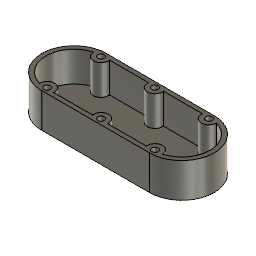
assembly_V.1 (Autodesk Fusion 360 archive; units mm, degrees)
design "robosoc_motor_case_without_motor_V.1"
part number: 2025-12-10-15-49-31-313
Autodesk Fusion 360 part; units mm, degrees
note: some values were not read from the file. Set by a fixed rule: the direction of a hole.
sketch "Sketch1" plane through (0, 0, 0) normal (0, 0, 1) x (1, 0, 0)
  line L0 (15, 0) -> (65, 0)
  line L1 (65, 30) -> (15, 30)
  arc A0 (15, 30) -> (0, 15) centre (15, 15) ccw
  arc A1 (0, 15) -> (15, 0) centre (15, 15) ccw
  arc A2 (80, 15) -> (65, 30) centre (65, 15) ccw
  arc A3 (65, 0) -> (80, 15) centre (65, 15) ccw
  line L2 (15, 15) -> (65, 15) construction
  line L3 (15, 15) -> (15, 27.5) construction
  line L4 (65, 15) -> (65, 27.5) construction
  line L5 (15, 27.5) -> (40, 27.5) construction
  circle A4 centre (15, 27.5) radius 1.5
  circle A5 centre (40, 27.5) radius 1.5
  circle A6 centre (65, 27.5) radius 1.5
  circle A7 centre (15, 2.5) radius 1.5
  circle A8 centre (40, 2.5) radius 1.5
  circle A9 centre (65, 2.5) radius 1.5
  circle A10 centre (65, 15) radius 2.5
  circle A11 centre (15, 15) radius 2.5
  point P0 (80, 0)
  point P1 (0, 30)
  dimension "d1" = 80
  dimension "d2" = 30
  dimension "d3" = 15
  dimension "d4" = 15
  dimension "d5" = 15
  dimension "d6" = 15
  dimension "d7" = 12.5
  dimension "d8" = 12.5
  dimension "d9" = 25
  dimension "d11" = 3
  dimension "d12" = 3
  dimension "d13" = 3
  dimension "d22" = 5
  dimension "d23" = 5
  constraint horizontal L0
  constraint horizontal L1
  constraint coincident P1 L1
  constraint tangent L1 A0
  constraint coincident origin L0
  constraint tangent L0 A1
  constraint coincident A0.end A1.start
  constraint tangent L1 A2
  constraint coincident P0 L0
  constraint tangent L0 A3
  constraint coincident A2.start A3.end
  constraint coincident A0.centre A1.centre
  constraint coincident A2.centre A3.centre
  constraint perpendicular L1 L3
  constraint perpendicular L2 L4
  constraint perpendicular L3 L5
  constraint coincident L3.end L5.start
  constraint coincident L5.end A5.centre
  constraint coincident L4.end A6.centre
  constraint symmetric L2 A4 A7
  constraint symmetric L2 A5 A8
  constraint symmetric L2 A6 A9
  constraint concentric A3 A10
  constraint concentric A1 A11
  measures "d1" distance of origin P0
  measures "d2" distance of origin P1
  measures "d3" radius of A0
  measures "d4" radius of A1
  measures "d5" radius of A2
  measures "d6" radius of A3
  measures "d7" distance of A0.centre L3.end
  measures "d8" distance of A2.centre L4.end
  measures "d9" distance of L3.end L5.end
  measures "d11" diameter of A4
  measures "d12" diameter of A5
  measures "d13" diameter of A6
  measures "d22" diameter of A10
  measures "d23" diameter of A11
extrude "Extrude1" add sketch "Sketch1" along normal blind 16 contours L0 L1 A0 A1 A2 A3 | A10 | A11
shell "Shell1" thickness 2 removed faces 1 at (23.6999, 18.8266, 16)
hole "Hole1" at (65, 27.5, 0) at (40, 27.5, 0) at (15, 27.5, 0) at (15, 2.5, 0) at (40, 2.5, 0) at (65, 2.5, 0) direction (0, 0, 1) diameter 4 depth 1 tip angle 180 countersink diameter 4.4 countersink angle 90
extrude "Extrude2" add sketch "Sketch1" against normal blind 4 draft -15 contours A10 | A11
equation "d23 = d22"

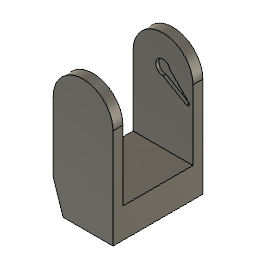
design "robosoc_leg_holder_V.1"
part number: 2025-12-04-10-49-25-755
Autodesk Fusion 360 part; units mm, degrees
sketch "Sketch1" plane through (0, 0, 0) normal (0, 1, 0) x (1, 0, 0)
  line L0 (5, 0) -> (30, 0)
  line L1 (30, 0) -> (30, -50)
  line L2 (0, -50) -> (0, -15)
  arc A0 (0, -50) -> (30, -50) centre (15, -50) ccw
  circle A1 centre (15, -50) radius 1.5
  line L3 (30, 0) -> (5, 0) construction
  line L4 (0, -15) -> (5, 0)
  line L5 (0, -15) -> (30, -15)
  dimension "d2" = 50
  dimension "d4" = 3
  dimension "d5" = 25
  dimension "d6" = 15
  dimension "d9" = 30
  constraint horizontal L0
  constraint vertical L1
  constraint vertical L2
  constraint concentric A0 A1
  constraint perpendicular L1 L3
  constraint perpendicular L1 L5
  measures "d2" distance of origin L2.start
  measures "d4" diameter of A1
  measures "d5" distance of L0.end L0.start
  measures "d6" distance of origin L2.end
  measures "d9" distance of L2.end L5.end
extrude "Extrude1" add sketch "Sketch1" along normal blind 5 contours L0 L1 L4 L5 | L1 L2 A0 L5 | A1
extrude "Extrude2" cut sketch "Sketch1" along normal blind 45 contours L0 L1 L4 L5
extrude "Extrude3" add sketch "Sketch1" along normal blind 22.5 contours L0 L1 L4 L5
mirror "Mirror1" about plane through (0, 22.5, 0) normal (0, 1, 0) of bodies 1 merged
hole "Hole2" at (15, 5, 50) direction (0, -1, 0) diameter 4.5 depth 4 tip angle 180
sketch "Sketch2" plane through (0, 40, 0) normal (0, -1, 0) x (1, 0, 0)
  line L0 (0, 15) -> (30, 15)
  line L1 (30, 15) -> (30, 50)
  arc A0 (30, 50) -> (0, 50) centre (15, 50) ccw
  line L2 (0, 50) -> (0, 15)
  line L3 (14.9863, 46.4) -> (18.4859, 50.8992) construction
  line L4 (15, 50) -> (28.0239, 39.8695) construction
  line L5 (18.4859, 50.8992) -> (27.951, 41.1812)
  line L6 (14.9863, 46.4) -> (26.7346, 39.6174)
  arc A1 (26.7346, 39.6174) -> (27.951, 41.1812) centre (27.2346, 40.4835) ccw
  arc A2 (18.4859, 50.8992) -> (14.9863, 46.4) centre (15, 50) ccw
  dimension "d24" = 7.2
  dimension "d25" = 2
  dimension "d26" = 5.7
  dimension "d28" = 16.5
  constraint concentric A0 A2
  constraint coincident A0.centre L4.start
  constraint coincident L4.end A1
  constraint tangent L5 A1
  constraint tangent L6 A1
  constraint perpendicular L3 L4
  constraint coincident A1.centre L4
  measures "d24" diameter of A2
  measures "d25" diameter of A1
  measures "d26" distance of L3.start L3.end
  measures "d28" distance of A0.centre L4.end
extrude "Extrude4" cut sketch "Sketch2" against normal blind 1.5 contours L5 L6 A1 A2
hole "Hole1" at (17.5, 22.5, 0) direction (0, 0, 1) diameter 19 depth 13 tip angle 180 countersink diameter 21 countersink angle 10

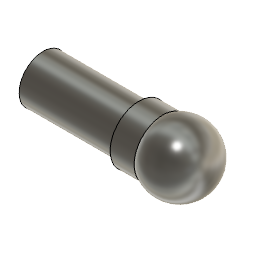
design "robosoc_leg_piece_V.1"
part number: 2025-12-04-11-27-23-377
Autodesk Fusion 360 part; units mm, degrees
sketch "Sketch1" plane through (0, 0, 0) normal (0, 0, 1) x (1, 0, 0)
  line L0 (0, 0) -> (50, 0)
  line L1 (50, 8) -> (50, 10)
  line L2 (40, 10) -> (0, 10)
  line L3 (0, 10) -> (0, 0)
  line L4 (50, 10) -> (40, 10) construction
  line L5 (50, 10) -> (50, 12)
  line L6 (50, 12) -> (40, 12)
  line L7 (40, 12) -> (40, 10)
  line L8 (50, 0) -> (57, 0) construction
  arc A0 (70.8924, 0) -> (50, 12) centre (57, 0) ccw
  arc A1 (69.2066, 0) -> (50, 10) centre (57, 0) ccw
  line L9 (50, 0) -> (70.8924, 0)
  line L10 (0, 0) -> (0, 8) construction
  line L11 (0, 8) -> (50, 8)
  line L12 (50, 8) -> (50, 10)
  dimension "d1" = 50
  dimension "d2" = 10
  dimension "d3" = 10
  dimension "d4" = 10
  dimension "d5" = 2
  dimension "d6" = 7
  dimension "d7" = 8
  dimension "d8" = 50
  constraint horizontal L0
  constraint vertical L1
  constraint horizontal L2
  constraint vertical L3
  constraint coincident L0.start L3.end
  constraint perpendicular L1 L4
  constraint vertical L5
  constraint horizontal L6
  constraint vertical L7
  constraint perpendicular L1 L8
  constraint coincident L8.end A0.centre
  constraint perpendicular L1 L9
  constraint perpendicular L0 L10
  constraint perpendicular L1 L11
  measures "d1" distance of L0.start L0.end
  measures "d2" distance of L0.start L2.end
  measures "d3" distance of L1.end L2.start
  measures "d4" distance of L2.start L1.end
  measures "d5" distance of L2.start L6.end
  measures "d6" distance of L0.end L8.end
  measures "d7" distance of L0.start L10.end
  measures "d8" distance of L10.end L1.start
revolve "Revolve1" add sketch "Sketch1" angle 360 about axis through (0, 0, 0) along (1, 0, 0) contours L1 L2 L3 L5 L6 L7 L11 L12 | L5 A0 A1 L9

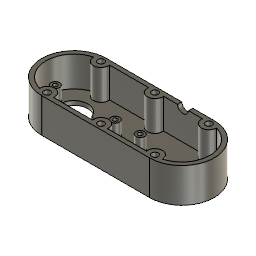
design "robosoc_motor_case_with_motor_V.1"
part number: 2025-12-10-15-49-31-313
Autodesk Fusion 360 part; units mm, degrees
sketch "Sketch1" plane through (0, 0, 0) normal (0, 0, 1) x (1, 0, 0)
  line L0 (15, 0) -> (65, 0)
  line L1 (65, 30) -> (15, 30)
  arc A0 (15, 30) -> (0, 15) centre (15, 15) ccw
  arc A1 (0, 15) -> (15, 0) centre (15, 15) ccw
  arc A2 (80, 15) -> (65, 30) centre (65, 15) ccw
  arc A3 (65, 0) -> (80, 15) centre (65, 15) ccw
  line L2 (15, 15) -> (65, 15) construction
  line L3 (15, 15) -> (15, 27.5) construction
  line L4 (65, 15) -> (65, 27.5) construction
  line L5 (15, 27.5) -> (40, 27.5) construction
  circle A4 centre (15, 27.5) radius 1.5
  circle A5 centre (40, 27.5) radius 1.5
  circle A6 centre (65, 27.5) radius 1.5
  circle A7 centre (15, 2.5) radius 1.5
  circle A8 centre (40, 2.5) radius 1.5
  circle A9 centre (65, 2.5) radius 1.5
  point P0 (80, 0)
  point P1 (0, 30)
  dimension "d1" = 80
  dimension "d2" = 30
  dimension "d3" = 15
  dimension "d4" = 15
  dimension "d5" = 15
  dimension "d6" = 15
  dimension "d7" = 12.5
  dimension "d8" = 12.5
  dimension "d9" = 25
  dimension "d11" = 3
  dimension "d12" = 3
  dimension "d13" = 3
  constraint horizontal L0
  constraint horizontal L1
  constraint coincident P1 L1
  constraint tangent L1 A0
  constraint coincident origin L0
  constraint tangent L0 A1
  constraint coincident A0.end A1.start
  constraint tangent L1 A2
  constraint coincident P0 L0
  constraint tangent L0 A3
  constraint coincident A2.start A3.end
  constraint coincident A0.centre A1.centre
  constraint coincident A2.centre A3.centre
  constraint perpendicular L1 L3
  constraint perpendicular L2 L4
  constraint perpendicular L3 L5
  constraint coincident L3.end L5.start
  constraint coincident L5.end A5.centre
  constraint coincident L4.end A6.centre
  constraint symmetric L2 A4 A7
  constraint symmetric L2 A5 A8
  constraint symmetric L2 A6 A9
  measures "d1" distance of origin P0
  measures "d2" distance of origin P1
  measures "d3" radius of A0
  measures "d4" radius of A1
  measures "d5" radius of A2
  measures "d6" radius of A3
  measures "d7" distance of A0.centre L3.end
  measures "d8" distance of A2.centre L4.end
  measures "d9" distance of L3.end L5.end
  measures "d11" diameter of A4
  measures "d12" diameter of A5
  measures "d13" diameter of A6
extrude "Extrude4" add sketch "Sketch1" along normal blind 2 contours A4 | A5 | A6 | A7 | A8 | A9 makes body 1 at (63.9526, 26.4262, 1.3333) makes body 2 at (41.4981, 2.4252, 1.3333) makes body 3 at (63.9526, 1.4262, 1.3333) makes body 4 at (38.9526, 26.4262, 1.3333) makes body 5 at (16.4981, 27.4252, 1.3333) makes body 6 at (16.4981, 2.4252, 1.3333)
extrude "Extrude1" add sketch "Sketch1" along normal blind 16 separate body makes body 7
shell "Shell1" thickness 2 removed faces 1 at (23.6999, 18.8266, 16) on bodies 7
sketch "Sketch2" plane through (0, 0, 2) normal (0, 0, 1) x (-1, 0, 0)
  arc A0 (-68.4999, -2.48) -> (-61.5359, -2) centre (-65, -2.5) ccw
  arc A1 (-68.4999, -2.48) -> (-68.4999, -27.52) centre (-65, -15) ccw
  arc A2 (-61.5359, -28) -> (-68.4999, -27.52) centre (-65, -27.5) ccw
  line L0 (-61.5359, -28) -> (-43.4641, -28)
  arc A3 (-36.5359, -28) -> (-43.4641, -28) centre (-40, -27.5) ccw
  line L1 (-36.5359, -28) -> (-18.4641, -28)
  arc A4 (-11.5001, -27.52) -> (-18.4641, -28) centre (-15, -27.5) ccw
  arc A5 (-11.5001, -27.52) -> (-11.5001, -2.48) centre (-15, -15) ccw
  arc A6 (-18.4641, -2) -> (-11.5001, -2.48) centre (-15, -2.5) ccw
  line L2 (-18.4641, -2) -> (-36.5359, -2)
  arc A7 (-43.4641, -2) -> (-36.5359, -2) centre (-40, -2.5) ccw
  line L3 (-43.4641, -2) -> (-61.5359, -2)
  line L4 (-15, -2.5) -> (-15, -27.5) construction
  arc A8 (-20.7264, -12.142) -> (-20.9934, -17.2449) centre (-21.0208, -14.6851) ccw
  arc A9 (-20.9934, -17.2449) -> (-20.7264, -12.142) centre (-15, -15) ccw
  arc A10 (-58.9129, -12.4127) -> (-58.8845, -17.522) centre (-64.7667, -15) ccw
  arc A11 (-58.8845, -17.522) -> (-58.9129, -12.4127) centre (-58.7336, -14.9664) ccw
  line L5 (-15, -15) -> (-34.1, -15) construction
  line L6 (-15, -15) -> (-6.3, -15) construction
  line L7 (-64.7667, -15) -> (-45.6667, -15) construction
  line L8 (-64.7667, -15) -> (-73.4667, -15) construction
  circle A12 centre (-6.3, -15) radius 1
  circle A13 centre (-34.1, -15) radius 1
  circle A14 centre (-73.4667, -15) radius 1
  circle A15 centre (-45.6667, -15) radius 1
  circle A16 centre (-34.1, -15) radius 2
  circle A17 centre (-6.3, -15) radius 2
  circle A18 centre (-45.6667, -15) radius 2
  circle A19 centre (-73.4667, -15) radius 2
  dimension "d17" = 12.8
  dimension "d18" = 12.8
  dimension "d19" = 5.12
  dimension "d20" = 5.12
  dimension "d22" = 19.1
  dimension "d23" = 8.7
  dimension "d24" = 19.1
  dimension "d25" = 8.7
  dimension "d26" = 2
  dimension "d27" = 2
  dimension "d29" = 2
  dimension "d31" = 2
  dimension "d32" = 1
  dimension "d33" = 1
  dimension "d34" = 1
  dimension "d35" = 1
  constraint coincident A6.centre L4.start
  constraint coincident A4.centre L4.end
  constraint concentric A5 A9
  constraint coincident A5.centre A9.centre
  constraint perpendicular L4 L5
  constraint perpendicular L4 L6
  constraint coincident A10.centre L7.start
  constraint parallel L1 L7
  constraint parallel L7 L8
  constraint coincident L6.end A12.centre
  constraint coincident L5.end A13.centre
  constraint coincident L8.end A14.centre
  constraint coincident L7.end A15.centre
  measures "d17" diameter of A9
  measures "d18" diameter of A10
  measures "d19" diameter of A8
  measures "d20" diameter of A11
  measures "d22" distance of A5.centre L5.end
  measures "d23" distance of A5.centre L6.end
  measures "d24" distance of A10.centre L7.end
  measures "d25" distance of A10.centre L8.end
  measures "d26" diameter of A12
  measures "d27" diameter of A13
  measures "d29" diameter of A14
  measures "d31" diameter of A15
  measures "d32" distance of A13
  measures "d33" distance of A12
  measures "d34" distance of A15
  measures "d35" distance of A14
extrude "Extrude2" cut sketch "Sketch2" against normal through all contours A8 A9 | A10 A11 bodies 7
extrude "Extrude3" add sketch "Sketch2" along normal blind 6.4 contours A16 | A17 | A18 | A19 bodies 7
sketch "Sketch3" plane through (0, 30, 0) normal (0, 1, 0) x (-1, 0, 0)
  line L0 (-65, 0) -> (-15, 0)
  line L1 (-15, 0) -> (-15, 16)
  line L2 (-15, 16) -> (-65, 16)
  line L3 (-65, 16) -> (-65, 0)
  line L4 (-65, 16) -> (-15, 16)
  line L5 (-65, 0) -> (-65, 16)
  line L6 (-65, 0) -> (-15, 0)
  line L7 (-15, 0) -> (-15, 16)
  line L8 (-65, 16) -> (-15, 16) construction
  line L9 (-65, 16) -> (-40, 16) construction
  line L10 (-65, 16) -> (-52.5, 16) construction
  circle A0 centre (-52.5, 16) radius 2.5
  dimension "d40" = 5
  constraint coincident L2.end L3.start
  constraint coincident L1.end L2.start
  constraint coincident L4 L9.end
  constraint midpoint L8 L9.end
  constraint midpoint L9 L10.end
  constraint coincident L10.end A0.centre
  measures "d40" diameter of A0
extrude "Extrude5" cut sketch "Sketch3" against normal up to surface (2 mm away) contours L2 L4 A0 picked at (-52.6854, 15.1876) bodies 7
equation "d3 = d4"
equation "d5 = d4"
equation "d6 = d4"
equation "d8 = d7"
equation "d11 = d12"
equation "d13 = d12"
equation "d17 = d18"
equation "d19 = d20"
equation "d20 = d18 / 2.5"
equation "d22 = d24"
equation "d23 = d25"
equation "d25 = 11 mm - 2.3 mm"
equation "d26 = d31"
equation "d27 = d31"
equation "d29 = d31"
equation "d32 = d34"
equation "d33 = d34"
equation "d35 = d34"

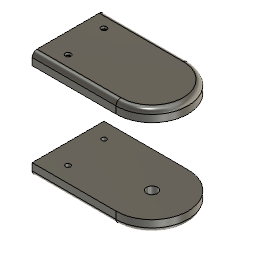
design "robosoc_body_holder_side_V.1"
part number: 2026-02-11-17-28-22-417
Autodesk Fusion 360 part; units mm, degrees
sketch "Sketch1" plane through (0, 0, 0) normal (0, 0, 1) x (1, 0, 0)
  line L0 (0, 0) -> (35, 0)
  line L1 (35, 30) -> (0, 30)
  line L2 (0, 30) -> (0, 0)
  circle A0 centre (35, 15) radius 2.25
  arc A1 (35, 0) -> (35, 30) centre (35, 15) ccw
  line L3 (15, 0) -> (15, 30)
  line L4 (15, 15) -> (0, 30) construction
  line L5 (7.5, 22.5) -> (7.5, 30) construction
  line L6 (7.5, 22.5) -> (0, 22.5) construction
  circle A2 centre (6.5, 23.5) radius 1
  circle A3 centre (8.5, 23.5) radius 1 construction
  circle A4 centre (8.5, 6.5) radius 1
  line L7 (15, 0) -> (0, 15) construction
  line L8 (7.5, 7.5) -> (7.5, 0) construction
  line L9 (7.5, 7.5) -> (15, 7.5) construction
  point P0 (40, 0)
  point P1 (15, 15)
  dimension "d1" = 30
  dimension "d7" = 35
  dimension "d8" = 35
  dimension "d9" = 4.5
  dimension "d14" = 2
  dimension "d36" = 2
  constraint horizontal L0
  constraint horizontal L1
  constraint vertical L2
  constraint coincident L0.start L2.end
  constraint coincident P0 L0
  constraint coincident A0.centre A1.centre
  constraint coincident L0 L3.start
  constraint coincident L1 L3.end
  constraint perpendicular L1 L3
  constraint midpoint L4 L5.start
  constraint coincident L1 L5.end
  constraint perpendicular L1 L5
  constraint coincident L2 L6.end
  constraint perpendicular L2 L6
  constraint coincident L4 A2.centre
  constraint tangent L5 A2
  constraint tangent L6 A2
  constraint symmetric L5 A2 A3
  constraint tangent L0 A1
  constraint midpoint L3 P1
  constraint coincident P1 L4.start
  constraint midpoint L2 L7.end
  constraint midpoint L7 L8.start
  constraint coincident L0 L8.end
  constraint perpendicular L0 L8
  constraint coincident L3 L9.end
  constraint perpendicular L3 L9
  constraint tangent A4 L9
  constraint tangent A4 L8
  measures "d1" distance of L0.start L1.end
  measures "d7" distance of L0.start L0.end
  measures "d8" distance of L1.end L1.start
  measures "d9" diameter of A0
  measures "d14" diameter of A2
  measures "d36" diameter of A4
extrude "Extrude1" add sketch "Sketch1" along normal blind 5 contours L0 L1 L2 L3 | L0 L1 A1 L3 | A0 | A2 | A4 makes body 1
hole "Hole1" at (8.5, 6.5, 0) at (6.5, 23.5, 0) direction (0, 0, 1) diameter 2 end through all counterbore diameter 2.3 counterbore depth 1 bodies 1
sketch "Sketch2" plane through (0, 0, 5) normal (0, 0, 1) x (-1, 0, 0)
  circle A0 centre (-8.5, -6.5) radius 1
  circle A1 centre (-6.5, -23.5) radius 1
  arc A2 (-35, 0) -> (-35, -30) centre (-35, -15) ccw
  line L0 (-35, -30) -> (0, -30)
  line L1 (0, -30) -> (0, 0)
  line L2 (0, 0) -> (-35, 0)
  circle A3 centre (-35, -15) radius 2.25
fillet "Fillet1" radius 2 3 edges at (17.5, 0, 0) (50, 15, 0) (17.5, 30, 0) on bodies 1
ref_plane "WorkPlane1" through (25, 15, 22.5) normal (0, 0, 1) x (1, 0, 0)
mirror "Mirror1" about plane through (25, 15, 22.5) normal (0, 0, 1) of bodies 1 makes body 2
extrude "Extrude2" cut sketch "Sketch2" against normal blind 4 contours A3 bodies 1
sketch "Sketch3" plane through (0, 0, 40) normal (0, 0, -1) x (1, 0, 0)
  circle A0 centre (8.5, -6.5) radius 1
  circle A1 centre (6.5, -23.5) radius 1
  arc A2 (35, -30) -> (35, 0) centre (35, -15) ccw
  line L0 (35, 0) -> (0, 0)
  line L1 (0, 0) -> (0, -30)
  line L2 (0, -30) -> (35, -30)
  line L3 (31.4, -14.9863) -> (24.6174, -26.7346)
  line L4 (35, -15) -> (24.8695, -28.0239) construction
  arc A3 (24.6174, -26.7346) -> (26.1812, -27.951) centre (25.4835, -27.2346) ccw
  line L5 (35.8992, -18.4859) -> (26.1812, -27.951)
  line L6 (31.4, -14.9863) -> (35.8992, -18.4859) construction
  arc A4 (35.8992, -18.4859) -> (31.4, -14.9863) centre (35, -15) ccw
  point P0 (35, -15)
  point P1 (35, -15)
  dimension "d30" = 2
  dimension "d31" = 5.7
  dimension "d32" = 16.5
  dimension "d33" = 7.2
  constraint coincident P1 P0
  constraint coincident L4.end A3
  constraint tangent A3 L5
  constraint tangent L3 A3
  constraint perpendicular L4 L6
  constraint coincident A3.centre L4
  measures "d30" diameter of A3
  measures "d31" distance of L3.start L5.start
  measures "d32" distance of L4.end P1
  measures "d33" diameter of A4
extrude "Extrude3" cut sketch "Sketch3" against normal blind 1.5 contours L3 A3 L5 A4 bodies 2
equation "d1 = breadth"
equation "breadth = 30 mm"
equation "length = 50 mm"
equation "d6 = 15 mm"
equation "d7 = length - d6"
equation "d8 = d7"
equation "d27 = ( 35 / 2 ) * 1 mm"
equation "d36 = d14"
